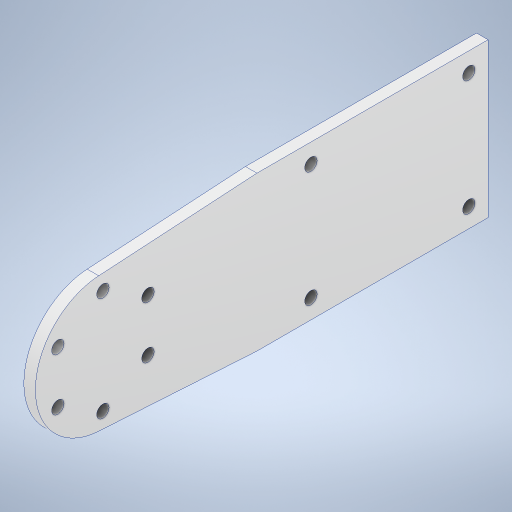
# Autodesk Inventor part: link6_plate1
Saved by Autodesk Inventor 2024 (Build 280153000, 153)
## iProperties
Created: 2024-12-13
Part Number: link6_plate1
Material: アルミニウム 6061
Document SubType Name: Modeling
Designer: hirek
Density: 2.7 g/cm^3
Appearance: アルミニウム - フラット
Mass: 37.9594 g
Surface Area: 106.915 cm^2
Volume: 14.059 cm^3
Author: hirek
Autodesk Inventor part; units mm, degrees
ref_plane "YZ Plane" through (0, 0, 0) normal (1, 0, 0) x (0, 1, 0)
ref_plane "XZ Plane" through (0, 0, 0) normal (0, 1, 0) x (-1, 0, 0)
ref_plane "XY Plane" through (0, 0, 0) normal (0, 0, 1) x (1, 0, 0)
sketch "スケッチ1" plane through (0, 0, 0) normal (1, 0, 0) x (0, 1, 0)
  line L0 (35, -40) -> (-5, -40)
  line L1 (-5, -40) -> (-5, -100)
  line L2 (-5, -100) -> (35, -100)
  line L3 (35, -100) -> (35, -40)
  circle A0 centre (15, 0) radius 17.5
  line L4 (35, -40) -> (32.4668, 1.0772)
  line L5 (-5, -40) -> (-2.4668, 1.0772)
  dimension "d1" = 40
  dimension "d2" = 60
  dimension "d54" = 35
  dimension "d55" = 20
  constraints: 12 end point, 2 parallel, 2 point on circle, 2 tangent, 1 centre point, 1 horizontal, 1 perpendicular
  measures "d1" distance of L2.end L1.end
  measures "d2" distance of L1.end L0.end
  measures "d54" diameter of A0
  measures "d55" distance from line of L3 A0.centre
extrude "押し出し1" add sketch "スケッチ1" along normal blind 3
sketch "スケッチ4" plane through (3, 0, 0) normal (1, 0, 0) x (0, 0, -1)
  line L0 (54, 30) -> (95, 30)
  line L1 (95, 30) -> (95, 0)
  line L2 (95, 0) -> (54, 0)
  line L3 (54, 0) -> (54, 30)
  line L4 (100, 35) -> (40, 35) projected
  line L5 (100, -5) -> (100, 35) projected
  point P0 (0, 0)
  dimension "d29" = 41
  dimension "d30" = 30
  dimension "d31" = 5
  dimension "d32" = 5
  constraints: 8 end point, 4 coincident, 2 parallel, 1 horizontal, 1 perpendicular
  measures "d29" distance of L1.end L2.end
  measures "d30" distance of L0.end L1.end
  measures "d31" distance between parallel lines of L0 L4
  measures "d32" distance between parallel lines of L5 L1
hole "穴2" at (3, 30, -54) at (3, 0, -54) at (3, 0, -95) at (3, 30, -95) direction (-1, 0, 0) diameter 3.2 end through all
sketch "スケッチ6" plane through (3, 0, 0) normal (1, 0, 0) x (0, 0, -1)
  arc A0 (-1.0772, 32.4668) -> (-1.0772, -2.4668) centre (0, 15) ccw projected
  circle A1 centre (0, 15) radius 13.5
  point P0 (0, 0)
  point P1 (0, 1.5)
  point P2 (11.6913, 8.25)
  point P3 (11.6913, 21.75)
  point P4 (0, 28.5)
  point P5 (-11.6913, 21.75)
  point P6 (-11.6913, 8.25)
  dimension "d56" = 27
  dimension "d59" = 360
  constraints: 1 coincident, 1 vertical alignment, 9 other
hole "穴4" at (3, 1.5, 0) at (3, 8.25, -11.6913) at (3, 21.75, -11.6913) at (3, 28.5, 0) at (3, 21.75, 11.6913) at (3, 8.25, 11.6913) direction (-1, 0, 0) diameter 3.2 end through all
